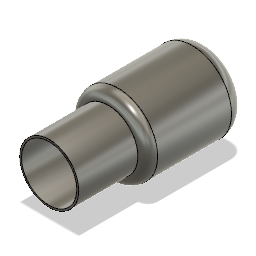
Bottle Revolve (Autodesk Fusion 360 design; units mm, degrees)
Autodesk Fusion 360 part; units mm, degrees
note: some values were not read from the file. Chosen so that the rebuilt part matches the saved one: which pieces of a blend or face edit are solid.
sketch "Sketch1" plane through (0, 0, 0) normal (0, 1, 0) x (1, 0, 0)
  line L0 (0, 0) -> (30, 0)
  line L1 (30, 0) -> (30, 60)
  line L2 (30, 60) -> (40, 60)
  line L3 (40, 60) -> (40, 160)
  line L4 (40, 160) -> (0, 160)
  line L5 (0, 160) -> (0, 0)
  dimension "d8" = 100
  dimension "d9" = 160
  dimension "d10" = 30
  constraint coincident L0.start L5.end
  constraint horizontal L0
  constraint perpendicular L0 L1
  constraint perpendicular L1 L2
  constraint perpendicular L0 L3
  constraint perpendicular L3 L4
  constraint perpendicular L0 L5
  measures "d8" distance of L2.end L3.end
  measures "d9" distance of L4.end L0.start
  measures "d10" distance of L0.start L0.end
revolve "Revolve1" add sketch "Sketch1" angle 360 about axis through (0, 0, -160) along (0, 0, 1)
fillet "Fillet1" radius 10 1 edges at (-37.2931, -14.4646, -60)
fillet "Fillet2" radius 15 1 edges at (-37.2931, -14.4646, -160)
shell "Shell1" thickness 2 removed faces 1 at (14.141, -6.0737, 0)
equation "overalheight = 160 mm"
equation "neckheight = 100 mm"
equation "fillet1 = 15 mm"
equation "fillet2 = 10 mm"
equation "fillet3 = 5 mm"
equation "diameter = 30 mm"
equation "wallthickness = 2 mm"
equation "d8 = neckheight"
equation "d9 = overalheight"
equation "d10 = diameter"
equation "d12 = fillet2"
equation "d13 = fillet1"
equation "d14 = wallthickness"
